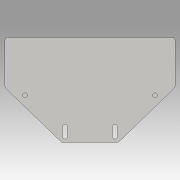
# Autodesk Inventor part: new pulley plate
Saved by Autodesk Inventor 2016 (Build 200138000, 138)
## iProperties
Created: 2015-11-24
Part Number: new pulley plate
Material: Generic
Document SubType Name: Modeling
Designer: Delta
Density: 1 g/cm^3
Appearance: Default
Author: Delta
Autodesk Inventor part; units mm, degrees
ref_plane "YZ Plane" through (0, 0, 0) normal (1, 0, 0) x (0, 1, 0)
ref_plane "XZ Plane" through (0, 0, 0) normal (0, 1, 0) x (-1, 0, 0)
ref_plane "XY Plane" through (0, 0, 0) normal (0, 0, 1) x (1, 0, 0)
sketch "Sketch1" plane through (0, 0, 0) normal (0, 0, 1) x (1, 0, 0)
  line L0 (0, 0) -> (215.9, 0)
  line L1 (215.9, 0) -> (215.9, 152.4)
  line L2 (215.9, 152.4) -> (0, 152.4)
  line L3 (0, 152.4) -> (0, 0)
  dimension "d0" = 215.9
  dimension "d1" = 152.4
  constraints: 8 end point, 2 parallel, 1 horizontal, 1 perpendicular
  measures "d0" distance of L2.end L1.end
  measures "d1" distance of L1.end L0.end
extrude "Extrusion1" add sketch "Sketch1" along normal blind 3.175
sketch "Sketch2" plane through (0, 0, 3.175) normal (0, 0, 1) x (1, 0, 0)
  line L0 (215.9, 152.4) -> (0, 152.4) construction
  line L1 (107.95, 152.4) -> (107.95, 0) construction
  line L2 (0, 0) -> (215.9, 0) projected
  point P0 (25.4, 59.8875)
  point P1 (76.2, 7.5)
  point P2 (190.5, 59.8875)
  point P3 (139.7, 7.5)
  dimension "d5" = 31.75
  dimension "d7" = 82.55
  dimension "d9" = 52.3875
  dimension "d10" = 7.5
  constraints: 2 end point, 2 symmetric about line, 1 midpoint, 1 vertical
  measures "d5" distance from line of L1 point (76.2, 7.5)
  measures "d7" distance from line of L1 point (25.4, 59.888)
  measures "d9" vertical distance of point (25.4, 59.888) point (76.2, 7.5)
  measures "d10" distance from line of L2 point (76.2, 7.5)
hole "Hole1" at (25.4, 59.8875, 3.175) at (76.2, 7.5, 3.175) at (190.5, 59.8875, 3.175) at (139.7, 7.5, 3.175) direction (0, 0, -1) diameter 6.35 end through all
sketch "Sketch3" plane through (0, 0, 3.175) normal (0, 0, 1) x (1, 0, 0)
  line L0 (215.9, 152.4) -> (0, 152.4) projected
  line L1 (107.95, 152.4) -> (107.95, 0)
  line L2 (0, 0) -> (215.9, 0) projected
  circle A0 centre (25.4, 59.8875) radius 3.175 projected
  circle A1 centre (76.2, 7.5) radius 3.175 projected
  line L3 (25.4, 59.8875) -> (76.2, 7.5) construction
  line L4 (0, 152.4) -> (0, 0) projected
  line L5 (0, 130.175) -> (0, 78.2462)
  line L6 (3.175, 133.35) -> (107.95, 133.35)
  line L7 (0, 133.35) -> (0, 125.3708)
  circle A2 centre (190.5, 59.8875) radius 3.175
  circle A3 centre (139.7, 7.5) radius 3.175
  line L8 (190.5, 59.8875) -> (139.7, 7.5) construction
  line L9 (215.9, 152.4) -> (215.9, 78.2462)
  line L10 (215.9, 133.35) -> (215.9, 76.9596)
  line L11 (212.725, 133.35) -> (107.95, 133.35)
  line L12 (215.9, 130.175) -> (215.9, 125.3708)
  line L13 (75.9713, 0) -> (107.95, 0)
  line L14 (139.9287, 0) -> (107.95, 0)
  line L15 (215.9, 0) -> (215.9, 152.4) projected
  line L16 (107.95, 59.7509) -> (194.45, 59.7509)
  line L17 (107.95, 59.7509) -> (194.45, 59.7509) construction
  line L18 (107.95, 59.7509) -> (21.45, 59.7509)
  line L19 (0, 0) -> (215.9, 0) projected
  line L20 (143.7779, 0) -> (215.9, 69.9366)
  line L21 (72.1221, 0) -> (0, 69.9366)
  line L22 (0, 152.4) -> (0, 0) projected
  line L23 (72.1221, 0) -> (107.95, 0)
  line L24 (3.175, 133.35) -> (0, 133.35)
  line L25 (212.725, 133.35) -> (215.9, 133.35)
  point P0 (74.6275, 0)
  point P1 (0, 76.9596)
  point P2 (77.9849, 0)
  dimension "d20" = 19.05
  dimension "d32" = 86.5
  dimension "d33" = 0
  dimension "d34" = 86.5
  dimension "d35" = 7.62
  dimension "d36" = 135.881
  dimension "d37" = 135.881
  dimension "d38" = 7.62
  dimension "d41" = 35.8279
  constraints: 40 end point, 22 point on line, 6 collinear, 5 symmetric about line, 3 horizontal, 2 centre point, 2 midpoint, 1 perpendicular, 1 vertical, 2 other
  measures "d20" distance between parallel lines of L6 L0
  measures "d32" distance of L16.start L16.end
  measures "d33" distance between parallel lines of L16 L17
  measures "d34" distance of L16.start L18.end
  measures "d35" distance from line of L20 L16.end
  measures "d36" angle of L20 L2
  measures "d37" angle of L21 L2
  measures "d38" distance from line of L21 L18.end
  measures "d41" distance from line of L1 L21.start
sketch "Sketch4" plane through (0, 0, 3.175) normal (0, 0, 1) x (1, 0, 0)
  arc A0 (79.3749, 20.1806) -> (73.0251, 20.1806) centre (76.2, 20.2) ccw
  circle A1 centre (76.2, 7.5) radius 3.175 projected
  circle A2 centre (76.2, 7.5) radius 3.175 projected
  line L0 (3.175, 133.35) -> (212.725, 133.35) projected
  line L1 (107.95, 133.35) -> (107.95, 0) construction
  line L2 (0, 0) -> (215.9, 0) projected
  arc A3 (142.8749, 20.176) -> (136.5251, 20.176) centre (139.7, 20.2) ccw
  arc A4 (73.0308, 7.5165) -> (79.3691, 7.4806) centre (76.2, 7.5) ccw
  circle A5 centre (139.7, 7.5) radius 3.175 projected
  arc A6 (136.5251, 7.5433) -> (142.8749, 7.5433) centre (139.7, 7.5) ccw
  line L3 (142.8749, 20.176) -> (142.8749, 7.476)
  circle A7 centre (139.7, 7.5) radius 3.175 projected
  line L4 (142.8749, 20.176) -> (155.5749, 20.176) construction
  line L5 (136.5251, 20.176) -> (136.5251, 7.476)
  line L6 (136.5251, 20.176) -> (149.2251, 20.176) construction
  line L7 (79.3749, 20.1806) -> (79.3749, 7.4806)
  line L8 (79.3749, 20.1806) -> (92.0749, 20.1806) construction
  line L9 (73.0251, 20.1806) -> (73.0309, 7.4806)
  line L10 (73.0251, 20.1806) -> (85.7251, 20.1806) construction
  line L11 (73.0251, 20.1806) -> (79.3749, 20.1806)
  line L12 (73.0309, 7.4806) -> (79.3749, 7.4806)
  line L13 (136.5251, 7.476) -> (142.8749, 7.476)
  line L14 (136.5251, 20.176) -> (142.8749, 20.176)
  point P0 (75.9713, 0)
  point P1 (139.9287, 0)
  point P2 (136.525, 7.4971)
  dimension "d29" = 6.35
  dimension "d30" = 12.7
  dimension "d44" = 90
  dimension "d45" = 90
  dimension "d46" = 90
  dimension "d48" = 12.7
  dimension "d49" = 12.7
  dimension "d50" = 12.7
  constraints: 26 end point, 9 point on circle, 4 centre point, 4 equal length, 4 horizontal, 4 point on line, 2 coincident, 2 midpoint, 2 parallel, 1 collinear, 1 symmetric about line, 3 other
  measures "d29" diameter of A0
  measures "d30" distance of A1.centre A0.centre
  measures "d44" angle of L3 L4
  measures "d45" angle of L5 L6
  measures "d46" angle of L7 L8
  measures "d48" distance of L9.start L9.end
  measures "d49" distance of L3.start L3.end
  measures "d50" distance of L5.start L5.end
extrude "Extrusion3" cut sketch "Sketch3" against normal blind 25.4 contours L9 L25 L11 L1 L0 | L1 L6 L24 L4 L0 | L2 L4 L21 | L20 L15 L2
extrude "Extrusion5" cut sketch "Sketch4" against normal blind 25.4
fillet "Fillet1" radius 3.175 6 edges at (0, 69.9366, 1.5875) (0, 133.35, 1.5875) (215.9, 133.35, 1.5875) (215.9, 69.9366, 1.5875) (143.7779, 0, 1.5875) (72.1221, 0, 1.5875)
equation "\"d34\" = d32"
equation "\"d37\" = d36"
equation "\"d38\" = d35"
equation "\"d48\" = d30"
equation "\"d49\" = d50"
body "Solid1"
